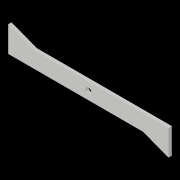
# Autodesk Inventor part: Front Weapon
Saved by Autodesk Inventor 2019 (Build 230136000, 136)
## iProperties
Created: 2017-12-11
Part Number: Front Weapon
Material: Generic
Document SubType Name: Modeling
Designer: rk_fe
Density: 1 g/cm^3
Appearance: Default
Author: rk_fe
Autodesk Inventor part; units mm, degrees
ref_plane "YZ Plane" through (0, 0, 0) normal (1, 0, 0) x (0, 1, 0)
ref_plane "XZ Plane" through (0, 0, 0) normal (0, 1, 0) x (-1, 0, 0)
ref_plane "XY Plane" through (0, 0, 0) normal (0, 0, 1) x (1, 0, 0)
sketch "Sketch1" plane through (0, 0, 0) normal (0, 0, 1) x (1, 0, 0)
  line L0 (0, 0) -> (508, 0)
  line L1 (508, 0) -> (508, 50.8)
  line L2 (508, 50.8) -> (0, 50.8)
  line L3 (0, 50.8) -> (0, 0)
  dimension "d0" = 508
  dimension "d1" = 50.8
  constraints: 8 end point, 2 parallel, 1 horizontal, 1 perpendicular
  measures "d0" distance of L1.end L2.end
  measures "d1" distance of L0.end L1.end
extrude "Extrusion1" add sketch "Sketch1" along normal blind 10.16
sketch "Sketch2" plane through (0, 0, 10.16) normal (0, 0, 1) x (1, 0, 0)
  line L0 (508, 50.8) -> (0, 50.8) projected
  line L1 (0, 50.8) -> (0, 81.28)
  line L2 (0, 81.28) -> (81.28, 50.8)
  line L3 (81.28, 50.8) -> (0, 50.8)
  line L4 (0, 0) -> (508, 0) projected
  line L5 (508, 0) -> (508, -30.48)
  line L6 (508, -30.48) -> (426.72, 0)
  dimension "d4" = 81.28
  dimension "d5" = 30.48
  dimension "d6" = 30.48
  dimension "d7" = 81.28
  constraints: 10 end point, 2 point on line, 2 vertical, 1 collinear
  measures "d4" distance of L0.end L2.end
  measures "d5" distance of L0.end L1.end
  measures "d6" distance of L4.end L5.end
  measures "d7" distance of L6.end L4.end
extrude "Extrusion2" add sketch "Sketch2" against normal blind 10.16
sketch "Sketch3" plane through (0, 0, 10.16) normal (0, 0, 1) x (1, 0, 0)
  line L0 (508, -30.48) -> (508, 50.8) projected
  line L1 (508, 0) -> (508, 50.8)
  line L2 (508, 25.4) -> (0, 25.4)
  line L3 (0, 81.28) -> (0, 0) projected
  circle A0 centre (254, 25.4) radius 9.525
  dimension "d10" = 19.05
  constraints: 4 end point, 2 midpoint, 2 point on line, 1 centre point, 1 collinear, 1 horizontal
  measures "d10" diameter of A0
extrude "Extrusion3" cut sketch "Sketch3" against normal blind 10.16
body "Solid1"
